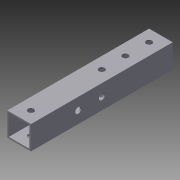
# Autodesk Inventor part: 1tube_6
Saved by Autodesk Inventor 2011 (Build 150239000, 239)
## iProperties
Created: 2013-01-16
Part Number: 1tube_6
Document SubType Name: Modeling
Designer: 917788
Density: 1 g/cm^3
Author: 917788
Autodesk Inventor part; units mm, degrees
ref_plane "YZ Plane" through (0, 0, 0) normal (1, 0, 0) x (0, 1, 0)
ref_plane "XZ Plane" through (0, 0, 0) normal (0, 1, 0) x (-1, 0, 0)
ref_plane "XY Plane" through (0, 0, 0) normal (0, 0, 1) x (1, 0, 0)
sketch "Sketch1" plane through (0, 0, 0) normal (0, 0, 1) x (1, 0, 0)
  line L0 (0, 0) -> (25.4, 0)
  line L1 (25.4, 0) -> (25.4, 25.4)
  line L2 (25.4, 25.4) -> (0, 25.4)
  line L3 (0, 25.4) -> (0, 0)
  line L4 (1.5875, 23.8125) -> (23.8125, 23.8125)
  line L5 (23.8125, 23.8125) -> (23.8125, 1.5875)
  line L6 (23.8125, 1.5875) -> (1.5875, 1.5875)
  line L7 (1.5875, 1.5875) -> (1.5875, 23.8125)
  dimension "d0" = 25.4
  dimension "d1" = 25.4
  dimension "d2" = 1.5875
  constraints: 16 end point, 4 parallel, 2 perpendicular, 1 horizontal, 3 other
  measures "d0" distance of L2.end L1.end
  measures "d1" distance of L1.end L0.end
  measures "d2" distance between parallel lines of L2 L4
extrude "Extrusion1" add sketch "Sketch1" against normal blind 152.4
sketch "Sketch2" plane through (0, 0, 0) normal (0, -1, 0) x (1, 0, 0)
  line L0 (0, -152.4) -> (25.4, -152.4) projected
  line L1 (0, 0) -> (25.4, 0) projected
  point P0 (12.7, -12.7)
  point P1 (12.7, -139.7)
  point P2 (12.7, -114.3)
  point P3 (12.7, -88.9)
  point P4 (12.7, -152.4)
  dimension "d5" = 25.4
  dimension "d6" = 25.4
  dimension "d7" = 12.7
  dimension "d8" = 12.7
  constraints: 4 vertical alignment, 1 midpoint
  measures "d5" distance of point (12.7, -114.3) point (12.7, -139.7)
  measures "d6" distance of point (12.7, -88.9) point (12.7, -114.3)
  measures "d7" distance from line of L0 point (12.7, -139.7)
  measures "d8" distance from line of L1 point (12.7, -12.7)
hole "Hole1" at (12.7, 0, -12.7) at (12.7, 0, -139.7) at (12.7, 0, -114.3) at (12.7, 0, -88.9) direction (0, 1, 0) diameter 6.35 depth 25.4 tip angle 118
sketch "Sketch3" plane through (0, 0, 0) normal (-1, 0, 0) x (0, 0, 1)
  line L0 (0, 25.4) -> (0, 0) projected
  point P0 (-44.45, 12.7)
  point P1 (-82.55, 12.7)
  dimension "d16" = 44.45
  dimension "d17" = 38.1
  measures "d16" distance from line of L0 point (-44.45, 12.7)
  measures "d17" distance of point (-44.45, 12.7) point (-82.55, 12.7)
hole "Hole2" at (0, 12.7, -44.45) at (0, 12.7, -82.55) direction (1, 0, 0) diameter 6.35 depth 25.4 tip angle 118
body "Solid1"
